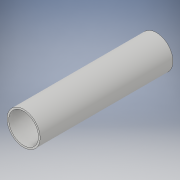
# Autodesk Inventor part: CAPTURE_3
Saved by Autodesk Inventor 2019 (Build 230136000, 136)
## iProperties
Created: 2019-07-24
Part Number: CAPTURE_3
Material: Generic
Document SubType Name: Modeling
Designer: afelepar
Density: 1 g/cm^3
Appearance: Default
Author: afelepar
Autodesk Inventor part; units mm, degrees
ref_plane "YZ Plane" through (0, 0, 0) normal (1, 0, 0) x (0, 1, 0)
ref_plane "XZ Plane" through (0, 0, 0) normal (0, 1, 0) x (-1, 0, 0)
ref_plane "XY Plane" through (0, 0, 0) normal (0, 0, 1) x (1, 0, 0)
sketch "Sketch1" plane through (0, 0, 0) normal (0, 0, 1) x (1, 0, 0)
  circle A0 centre (0, 0) radius 3.12
  dimension "d0" = 6.24
  constraints: 1 centre point, 1 coincident
  measures "d0" diameter of A0
extrude "Extrusion1" add sketch "Sketch1" along normal blind 25.02
sketch "Sketch2" plane through (0, 0, 25.02) normal (0, 0, 1) x (1, 0, 0)
  circle A0 centre (0, 0) radius 2.8
  dimension "d3" = 5.6
  constraints: 1 centre point, 1 coincident
  measures "d3" diameter of A0
extrude "Extrusion2" cut sketch "Sketch2" against normal through all
body "Solid1"
